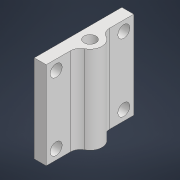
# Autodesk Inventor part: Piston Mount
Saved by Autodesk Inventor 2022 (Build 260153000, 153)
## iProperties
Created: 2022-09-18
Part Number: Piston Mount
Material: Generic
Document SubType Name: Modeling
Designer: robpl
Density: 1 g/cm^3
Appearance: Default
Author: robpl
Autodesk Inventor part; units mm, degrees
ref_plane "YZ Plane" through (0, 0, 0) normal (1, 0, 0) x (0, 1, 0)
ref_plane "XZ Plane" through (0, 0, 0) normal (0, 1, 0) x (-1, 0, 0)
ref_plane "XY Plane" through (0, 0, 0) normal (0, 0, 1) x (1, 0, 0)
sketch "Sketch1" plane through (0, 0, 0) normal (1, 0, 0) x (0, 1, 0)
  line L0 (0, 0) -> (44, 0)
  line L1 (44, 0) -> (44, 44)
  line L2 (44, 44) -> (0, 44)
  line L3 (0, 44) -> (0, 0)
  dimension "d2" = 44
  constraints: 8 end point, 2 parallel, 2 perpendicular, 1 horizontal
  measures "d2" distance of L2.end L0.start
extrude "Extrusion1" add sketch "Sketch1" along normal blind 12
sketch "Sketch2" plane through (12, 0, 0) normal (1, 0, 0) x (0, 0, -1)
  line L0 (-44, 44) -> (-44, 0) projected
  line L1 (0, 44) -> (-44, 44) projected
  point P0 (0, 0)
  point P1 (-5, 5)
  point P2 (-39, 5)
  point P3 (-39, 39)
  point P4 (-5, 39)
  dimension "d3" = 5
  dimension "d4" = 5
  dimension "d5" = 5
  dimension "d6" = 5
  constraints: 2 horizontal alignment, 2 vertical alignment
  measures "d3" horizontal distance of point (0, 0) point (-5, 5)
  measures "d4" horizontal distance of point (-5, 5) point (0, 0)
  measures "d5" distance from line of point (-39, 5) L0
  measures "d6" distance from line of L1 point (-39, 39)
hole "Hole1" at (12, 5, 5) at (12, 5, 39) at (12, 39, 39) at (12, 39, 5) direction (-1, 0, 0) diameter 6 end through all
sketch "Sketch3" plane through (0, 44, 44) normal (0, 1, 0) x (1, 0, 0)
  line L0 (0, 0) -> (12, 0) projected
  point P0 (0, 44)
  point P1 (6, 22)
  dimension "d14" = 6
  dimension "d15" = 22
  measures "d14" horizontal distance of point (0, 44) point (6, 22)
  measures "d15" distance from line of L0 point (6, 22)
hole "Hole2" at (6, 44, 22) direction (0, -1, 0) diameter 6 end through all
sketch "Sketch4" plane through (0, 44, 44) normal (0, 1, 0) x (1, 0, 0)
  circle A0 centre (6, 22) radius 3 projected
  line L0 (0, 44) -> (0, 0) projected
  line L1 (0, 0) -> (12, 0) projected
  line L2 (12, 44) -> (12, 0) projected
  line L3 (0, 44) -> (12, 44) projected
  circle A1 centre (6, 22) radius 3 projected
  circle A2 centre (6, 22) radius 6
  line L4 (0, 44) -> (12, 44) projected
  line L5 (0, 0) -> (12, 0) projected
  line L6 (12, 44) -> (12, 0)
  line L7 (12, 0) -> (6, 0)
  line L8 (6, 0) -> (6, 44)
  line L9 (6, 44) -> (12, 44)
  line L10 (12, 44) -> (12, 0) projected
  point P0 (6, 28)
  point P1 (12, 22)
  point P2 (6, 16)
  point P3 (6, 0)
  dimension "d23" = 6
  constraints: 8 end point, 2 parallel, 2 perpendicular, 1 centre point, 1 coincident, 1 tangent
  measures "d23" distance between parallel lines of L8 L2
extrude "Extrusion2" cut sketch "Sketch4" against normal blind 50 contours L8 L3 L2 A2 | A2 L2 L1 L8
fillet "Fillet1" radius 5 2 edges at (6, 22, 28) (6, 22, 16)
equation "\"d4\" = d3"
equation "\"d5\" = d3"
equation "\"d6\" = d3"
body "Solid1"
